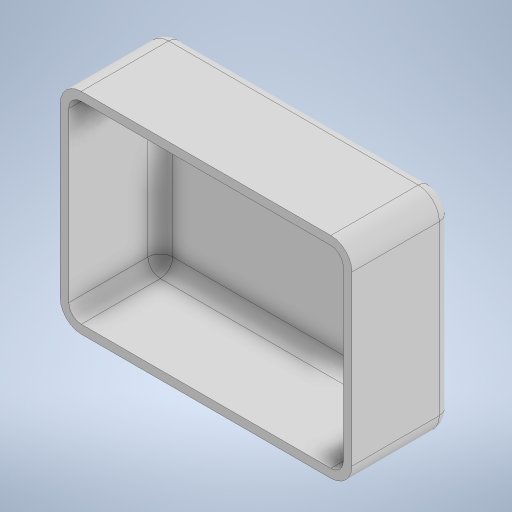
# Autodesk Inventor part: Корпус НАСУ
Saved by Autodesk Inventor 2023.1 (Build 271208000, 208)
## iProperties
Created: 2023-02-12
Part Number: Корпус НАСУ
Material: Типовые
Document SubType Name: Modeling
Designer: User
Density: 1 g/cm^3
Appearance: По умолчанию
Author: User
Autodesk Inventor part; units mm, degrees
ref_plane "YZ Plane" through (0, 0, 0) normal (1, 0, 0) x (0, 1, 0)
ref_plane "XZ Plane" through (0, 0, 0) normal (0, 1, 0) x (-1, 0, 0)
ref_plane "XY Plane" through (0, 0, 0) normal (0, 0, 1) x (1, 0, 0)
sketch "Эскиз1" plane through (0, 0, 0) normal (0, 0, 1) x (1, 0, 0)
  line L0 (-150, 116) -> (150, 116)
  line L1 (165, 101) -> (165, -101)
  line L2 (150, -116) -> (-150, -116)
  line L3 (-165, -101) -> (-165, 101)
  line L4 (-252.8728, 0) -> (252.8728, 0) projected
  line L5 (0, -184.2728) -> (0, 184.2728) projected
  arc A0 (-150, 116) -> (-165, 101) centre (-150, 101) ccw
  arc A1 (165, 101) -> (150, 116) centre (150, 101) ccw
  arc A2 (150, -116) -> (165, -101) centre (150, -101) ccw
  arc A3 (-165, -101) -> (-150, -116) centre (-150, -101) ccw
  line L6 (-175.3693, 101) -> (-175.3693, -101)
  arc A4 (-175.3693, -101) -> (-150, -126.3693) centre (-150, -101) ccw
  line L7 (-150, -126.3693) -> (150, -126.3693)
  arc A5 (150, -126.3693) -> (175.3693, -101) centre (150, -101) ccw
  line L8 (175.3693, -101) -> (175.3693, 101)
  arc A6 (175.3693, 101) -> (150, 126.3693) centre (150, 101) ccw
  line L9 (150, 126.3693) -> (-150, 126.3693)
  arc A7 (-150, 126.3693) -> (-175.3693, 101) centre (-150, 101) ccw
  point P0 (0, 0)
  dimension "d0" = 232
  dimension "d1" = 330
  dimension "d2" = 15
  constraints: 16 end point, 16 point on circle, 8 centre point, 8 tangent, 4 parallel, 3 equal radius, 2 perpendicular, 1 horizontal, 9 other
  measures "d0" distance between parallel lines of L2 L0
  measures "d1" distance between parallel lines of L3 L1
  measures "d2" radius of A0
extrude "Выдавливание1" add sketch "Эскиз1" along normal blind 110 contours A0 L3 L4 L6 A7 L9 L5 L0 | L5 L9 A6 L8 L4 L1 A1 L0 | L3 A3 L2 L5 L7 A4 L6 L4 | L4 L8 A5 L7 L5 L2 A2 L1
sketch "Эскиз2" plane through (0, 0, 0) normal (0, 0, -1) x (-1, 0, 0)
  line L0 (150, -126.3693) -> (-150, -126.3693) projected
  arc A0 (150, -126.3693) -> (175.3693, -101) centre (150, -101) ccw projected
  line L1 (175.3693, 101) -> (175.3693, -101) projected
  arc A1 (175.3693, 101) -> (150, 126.3693) centre (150, 101) ccw projected
  line L2 (-150, 126.3693) -> (150, 126.3693) projected
  arc A2 (-150, 126.3693) -> (-175.3693, 101) centre (-150, 101) ccw projected
  line L3 (-175.3693, -101) -> (-175.3693, 101) projected
  arc A3 (-175.3693, -101) -> (-150, -126.3693) centre (-150, -101) ccw projected
  point P0 (0, 0)
extrude "Выдавливание2" add sketch "Эскиз2" along normal blind 10
fillet "Сопряжение1" radius 15 8 edges at (-167.9388, -118.9388, -10) (-175.3693, 0, -10) (-167.9388, 118.9388, -10) (0, 126.3693, -10) (167.9388, 118.9388, -10) (175.3693, 0, -10) (167.9388, -118.9388, -10) (0, -126.3693, -10)
fillet "Сопряжение2" radius 15 8 edges at (160.6066, 111.6066, 0) (165, 0, 0) (160.6066, -111.6066, 0) (0, -116, 0) (-160.6066, -111.6066, 0) (-165, 0, 0) (-160.6066, 111.6066, 0) (0, 116, 0)
